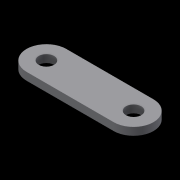
# Autodesk Inventor part: BackSideConnector
Saved by Autodesk Inventor 2015 (Build 190159000, 159)
## iProperties
Created: 2015-05-13
Part Number: BackSideConnector
Material: Generic
Document SubType Name: Modeling
Designer: Val
Density: 1 g/cm^3
Appearance: Default
Author: Val
Autodesk Inventor part; units mm, degrees
ref_plane "YZ Plane" through (0, 0, 0) normal (1, 0, 0) x (0, 1, 0)
ref_plane "XZ Plane" through (0, 0, 0) normal (0, 1, 0) x (-1, 0, 0)
ref_plane "XY Plane" through (0, 0, 0) normal (0, 0, 1) x (1, 0, 0)
sketch "Base" plane through (0, 0, 0) normal (0, 0, 1) x (1, 0, 0)
  circle A0 centre (0, 0) radius 7.75
  line L0 (0, 0) -> (-34, 0) construction
  circle A1 centre (-34, 0) radius 7.75
  circle A2 centre (0, 0) radius 3
  circle A3 centre (-34, 0) radius 3
  line L1 (-34, 7.75) -> (0, 7.75)
  line L2 (-34, -7.75) -> (0, -7.75)
  dimension "d0" = 15.5
  dimension "d1" = 34
  dimension "d3" = 6
  constraints: 6 end point, 4 centre point, 4 coincident, 4 point on circle, 4 tangent, 2 equal radius, 1 horizontal
  measures "d0" diameter of A0
  measures "d1" distance of L0.start L0.end
  measures "d3" diameter of A2
extrude "BaseFeature" add sketch "Base" along normal blind 3
